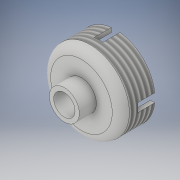
# Autodesk Inventor part: input
Saved by Autodesk Inventor 2019 (Build 230136000, 136)
## iProperties
Created: 2020-03-31
Part Number: input
Material: Generic
Document SubType Name: Modeling
Designer: Bishoy
Density: 1 g/cm^3
Appearance: Default
Author: Bishoy
Autodesk Inventor part; units mm, degrees
ref_plane "XY Plane" through (0, 0, 0) normal (0, 0, 1) x (1, 0, 0)
sketch "Sketch1" plane through (0, 0, 0) normal (0, 0, 1) x (1, 0, 0)
  circle A0 centre (0, 0) radius 41
  circle A1 centre (0, 0) radius 12.5
  circle A2 centre (0, 0) radius 46
  dimension "d0" = 82
  dimension "d1" = 25
  dimension "d2" = 92
  constraints: 3 centre point, 3 coincident
  measures "d0" diameter of A0
  measures "d1" diameter of A1
  measures "d2" diameter of A2
extrude "Extrusion1" add sketch "Sketch1" along normal blind 40 contours A0 | A2
fillet "Fillet1" radius 10 1 edges at (-46, 0, 40)
extrude "Extrusion2" cut sketch "Sketch1" along normal blind 33 contours A0
sketch "Sketch2" plane through (0, 0, 40) normal (0, 0, 1) x (1, 0, 0)
  circle A0 centre (0, 0) radius 17.5
  dimension "d8" = 35
  constraints: 1 centre point, 1 coincident
  measures "d8" diameter of A0
extrude "Extrusion3" add sketch "Sketch2" along normal blind 20
extrude "Extrusion4" cut sketch "Sketch1" along normal blind 118.5 contours A1
thread "Thread1" size "M95x6" class "6g" standard "ANSI Metric M Profile" full length
ref_plane "Work Plane1" through (0, -46, 0) normal (0, 1, 0) x (-1, 0, 0)
ref_plane "Work Plane2" through (46, 0, 0) normal (1, 0, 0) x (0, 1, 0)
sketch "Sketch3" plane through (0, -46, 0) normal (0, 1, 0) x (-1, 0, 0)
  line L0 (5, 20) -> (-5, 20)
  line L1 (-5, 20) -> (-5, -20)
  line L2 (-5, -20) -> (5, -20)
  line L3 (5, -20) -> (5, 20)
  line L4 (5, 20) -> (-5, -20) construction
  line L5 (-5, 20) -> (5, -20) construction
  point P0 (0, 0)
  dimension "d15" = 10
  dimension "d16" = 40
  constraints: 12 end point, 2 midpoint, 2 parallel, 1 horizontal, 1 perpendicular
  measures "d15" distance of L2.end L1.end
  measures "d16" distance of L1.end L0.end
extrude "Extrusion5" cut sketch "Sketch3" along normal blind 154.5
sketch "Sketch4" plane through (46, 0, 0) normal (1, 0, 0) x (0, 1, 0)
  line L0 (-5, 20) -> (5, 20)
  line L1 (5, 20) -> (5, -20)
  line L2 (5, -20) -> (-5, -20)
  line L3 (-5, -20) -> (-5, 20)
  line L4 (-5, 20) -> (5, -20) construction
  line L5 (5, 20) -> (-5, -20) construction
  point P0 (0, 0)
  dimension "d19" = 10
  dimension "d20" = 40
  constraints: 12 end point, 2 midpoint, 2 parallel, 1 horizontal, 1 perpendicular
  measures "d19" distance of L1.end L2.end
  measures "d20" distance of L0.end L1.end
extrude "Extrusion6" cut sketch "Sketch4" against normal blind 154.5
body "Solid1"
